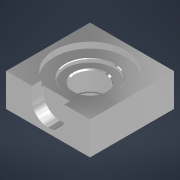
# Autodesk Inventor part: Soporte
Saved by Autodesk Inventor 2022 (Build 260153000, 153)
## iProperties
Created: 2021-09-20
Part Number: Soporte
Material: Aluminum 6061
Document SubType Name: Modeling
Designer: Andres
Density: 2.7 g/cm^3
Appearance: Aluminum - Flat
Author: Andres
Autodesk Inventor part; units mm, degrees
ref_plane "YZ Plane" through (0, 0, 0) normal (1, 0, 0) x (0, 1, 0)
ref_plane "XZ Plane" through (0, 0, 0) normal (0, 1, 0) x (-1, 0, 0)
ref_plane "XY Plane" through (0, 0, 0) normal (0, 0, 1) x (1, 0, 0)
sketch "Sketch1" plane through (0, 0, 0) normal (0, 1, 0) x (-1, 0, 0)
  circle A0 centre (0, 0) radius 60
  line L0 (-70, 70) -> (70, 70)
  line L1 (70, 70) -> (70, -70)
  line L2 (70, -70) -> (-70, -70)
  line L3 (-70, -70) -> (-70, 70)
  line L4 (-70, 70) -> (70, -70) construction
  line L5 (70, 70) -> (-70, -70) construction
  circle A1 centre (0, 0) radius 23
  dimension "d0" = 120
  dimension "d1" = 140
  dimension "d2" = 140
  dimension "Db" = 46
  constraints: 12 end point, 2 centre point, 2 coincident, 2 midpoint, 2 parallel, 1 horizontal, 1 perpendicular
  measures "d0" diameter of A0
  measures "d1" distance of L1.end L2.end
  measures "d2" distance of L0.end L1.end
  measures "Db" diameter of A1
extrude "Extrusion1" add sketch "Sketch1" along normal blind 10 contours L0 L1 L2 L3
extrude "Extrusion2" add sketch "Sketch1" against normal blind 45 contours A0 | L0 L1 L2 L3
sketch "Sketch2" plane through (0, 0, 0) normal (0, 1, 0) x (1, 0, 0)
  circle A0 centre (0, 0) radius 26
  circle A1 centre (0, 0) radius 23 projected
  dimension "d8" = 52
  constraints: 1 centre point, 1 coincident
  measures "d8" diameter of A0
extrude "Extrusion3" cut sketch "Sketch2" against normal blind 38
sketch "Plate Mounting Holes" plane through (-70, 10, 70) normal (0, 0, 1) x (1, 0, 0)
  line L0 (140, -55) -> (140, 0) construction
  line L1 (0, 0) -> (140, 0) construction
  line L2 (0, -55) -> (0, 0) construction
  line L3 (140, -55) -> (0, -55) construction
  line L4 (30, -50) -> (110, -50) construction
  line L5 (110, -50) -> (110, -5) construction
  line L6 (110, -5) -> (30, -5) construction
  line L7 (30, -5) -> (30, -50) construction
  line L8 (30, -50) -> (110, -5) construction
  line L9 (110, -50) -> (30, -5) construction
  point P0 (70, -10)
  point P1 (70, -27.5)
  point P2 (70, -27.5)
  point P3 (70, 0)
  dimension "d14" = 5
  dimension "d15" = 5
  dimension "d16" = 80
  constraints: 12 end point, 4 coincident, 4 midpoint, 2 parallel, 1 horizontal, 1 perpendicular, 1 vertical alignment
  measures "d14" distance between parallel lines of L1 L6
  measures "d15" distance between parallel lines of L3 L4
  measures "d16" distance between parallel lines of L5 L7
sketch "PlateHole" plane through (-70, 10, 70) normal (0, 0, 1) x (1, 0, 0)
  line L0 (43, -50) -> (97, -50)
  line L1 (97, -50) -> (97, 0)
  line L2 (97, 0) -> (43, 0)
  line L3 (43, 0) -> (43, -50)
  line L4 (43, -50) -> (97, 0) construction
  line L5 (97, -50) -> (43, 0) construction
  line L6 (140, -55) -> (0, -55) projected
  line L7 (0, 0) -> (140, 0) projected
  circle A0 centre (70, -20) radius 27
  point P0 (70, -10)
  point P1 (70, -25)
  point P2 (70, -27.5)
  point P3 (70, -25)
  point P4 (43, -20)
  point P5 (97, -20)
  dimension "d18" = 5
  dimension "d24" = 20
  dimension "d25" = 54
  constraints: 12 end point, 3 midpoint, 2 parallel, 2 tangent, 1 centre point, 1 collinear, 1 horizontal, 1 perpendicular, 1 vertical alignment
  measures "d18" distance between parallel lines of L6 L0
  measures "d24" distance from line of L7 A0.centre
  measures "d25" distance between parallel lines of L1 L3
sketch "Sketch7" plane through (0, 0, 0) normal (0, 1, 0) x (1, 0, 0)
  circle A0 centre (0, 0) radius 26 projected
  circle A1 centre (0, 0) radius 26 projected
  circle A2 centre (0, 0) radius 40
  dimension "d19" = 80
  constraints: 1 centre point, 1 coincident
  measures "d19" diameter of A2
extrude "Extrusion4" cut sketch "Sketch7" against normal blind 6
extrude "Extrusion5" cut sketch "PlateHole" against normal blind 20 contours L3 L2 A0 | A0 L2 | A0 L2 L1 picked at (79.2183, -12.2454)
chamfer "Chamfer2" distance 2 angle 45 1 edges at (-26, -6, 0)
chamfer "Chamfer3" distance 1 angle 45 1 edges at (-40, 0, 0)
equation "\"d15\" = d14"
body "Solid1"
